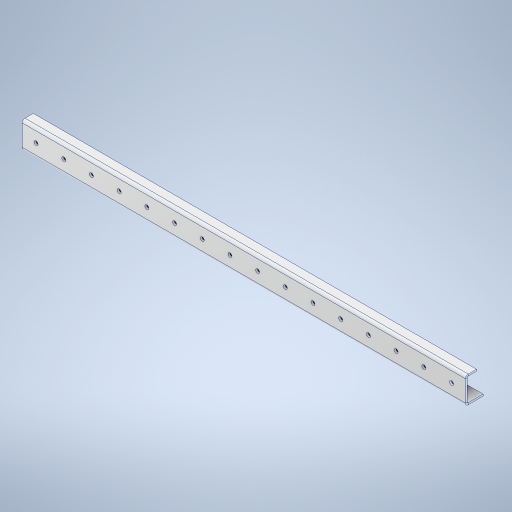
# Autodesk Inventor part: Gantry Stiffener
Saved by Autodesk Inventor 2024 (Build 280153000, 153)
## iProperties
Created: 2023-06-16
Part Number: Gantry Stiffener
Material: Aluminum 6061
Document SubType Name: Sheet Metal
Designer: Ishaan
Density: 2.7 g/cm^3
Appearance: Aluminum - Flat
Sheet Metal Rule: SendCutSend_Alu_1-16
Author: Ishaan
Autodesk Inventor part; units mm, degrees
ref_plane "YZ Plane" through (0, 0, 0) normal (1, 0, 0) x (0, 1, 0)
ref_plane "XZ Plane" through (0, 0, 0) normal (0, 1, 0) x (-1, 0, 0)
ref_plane "XY Plane" through (0, 0, 0) normal (0, 0, 1) x (1, 0, 0)
sketch "Sketch1" plane through (0, 0, 0) normal (0, 0, 1) x (1, 0, 0)
  line L0 (200, -12) -> (-200, -12)
  line L1 (-200, -12) -> (-200, 12)
  line L2 (-200, 12) -> (200, 12)
  line L3 (200, 12) -> (200, -12)
  line L4 (200, -12) -> (-200, 12) construction
  line L5 (-200, -12) -> (200, 12) construction
  point P0 (0, 0)
  dimension "d69" = 400
  dimension "d70" = 24
  constraints: 12 end point, 2 midpoint, 2 parallel, 1 horizontal, 1 perpendicular
  measures "d69" distance of L1.end L2.end
  measures "d70" distance of L0.end L1.end
extrude "Plate4" add sketch "Sketch1" along normal blind 1.6002
sketch "Sketch6" plane through (200, 10.3998, 1.6002) normal (0, 1, 0) x (-1, 0, 0)
  line L0 (400, 0) -> (0, 0)
  line L1 (0, 0) -> (0, -10)
  line L2 (0, -10) -> (400, -10)
  line L3 (400, -10) -> (400, 0)
  constraints: 6 end point, 1 horizontal, 1 perpendicular, 1 vertical
edge flange "Flange3" height 10 angle 90 thickness 1.6002 bend radius 0.889 thickness toward (0, 1, 0) relief tear relief width 1.6002 relief depth 0.8001 edges at (0, 12, 0) wall of the first edge with corners at (-200, 10.3998, 1.6002) (200, 10.3998, 1.6002) (200, 10.3998, -8.3998) (-200, 10.3998, -8.3998)
bend "Bend3"
corner "Corner3"
sketch "Sketch7" plane through (-200, -10.3998, 1.6002) normal (0, -1, 0) x (1, 0, 0)
  line L0 (400, 0) -> (0, 0)
  line L1 (0, 0) -> (0, -16)
  line L2 (0, -16) -> (400, -16)
  line L3 (400, -16) -> (400, 0)
  constraints: 6 end point, 1 horizontal, 1 perpendicular, 1 vertical
edge flange "Flange4" height 16 angle 90 thickness 1.6002 bend radius 0.889 thickness toward (0, -1, 0) relief tear relief width 1.6002 relief depth 0.8001 edges at (0, -12, 0) wall of the first edge with corners at (200, -10.3998, 1.6002) (-200, -10.3998, 1.6002) (-200, -10.3998, -14.3998) (200, -10.3998, -14.3998)
bend "Bend4"
corner "Corner4"
sketch "Sketch8" plane through (0, 0, 1.6002) normal (0, 0, 1) x (1, 0, 0)
  line L0 (-280, 0) -> (280, 0) construction
  line L1 (-187.5, 0) -> (187.5, 0) construction
  point P0 (0, 0)
  point P1 (-162.5, 0)
  point P2 (-137.5, 0)
  point P3 (-112.5, 0)
  point P4 (-87.5, 0)
  point P5 (-62.5, 0)
  point P6 (-37.5, 0)
  point P7 (-12.5, 0)
  point P8 (12.5, 0)
  point P9 (37.5, 0)
  point P10 (62.5, 0)
  point P11 (87.5, 0)
  point P12 (112.5, 0)
  point P13 (137.5, 0)
  point P14 (162.5, 0)
  dimension "d94" = 25
  constraints: 2 end point, 2 horizontal, 1 midpoint, 15 other
  measures "d94" distance of L1.start point (-162.5, 0)
hole "Hole3" at (-187.5, 0, 1.6002) at (-162.5, 0, 1.6002) at (-137.5, 0, 1.6002) at (-112.5, 0, 1.6002) at (-87.5, 0, 1.6002) at (-62.5, 0, 1.6002) at (-37.5, 0, 1.6002) at (-12.5, 0, 1.6002) at (12.5, 0, 1.6002) at (37.5, 0, 1.6002) at (62.5, 0, 1.6002) at (87.5, 0, 1.6002) at (112.5, 0, 1.6002) at (137.5, 0, 1.6002) at (162.5, 0, 1.6002) at (187.5, 0, 1.6002) direction (0, 0, -1) diameter 3.5 end through all
sketch "Sketch9" plane through (-200, -12, -14.3998) normal (0, -1, 0) x (1, 0, 0)
  line L0 (110, -6) -> (90, -6)
  line L1 (90, -6) -> (90, 13.5)
  line L2 (90, 13.5) -> (110, 13.5)
  line L3 (110, 13.5) -> (110, -6)
  line L4 (110, -6) -> (90, 13.5) construction
  line L5 (90, -6) -> (110, 13.5) construction
  line L6 (100, -4.3329) -> (93, -0.2915)
  line L7 (93, -0.2915) -> (93, 7.7915)
  line L8 (93, 7.7915) -> (100, 11.8329)
  line L9 (100, 11.8329) -> (107, 7.7915)
  line L10 (107, 7.7915) -> (107, -0.2915)
  line L11 (107, -0.2915) -> (100, -4.3329)
  line L12 (93, 7.7915) -> (100, 3.75)
  line L13 (100, 3.75) -> (107, 7.7915)
  line L14 (93, 2.4028) -> (100, -1.6386)
  line L15 (100, -1.6386) -> (107, 2.4028)
  line L16 (107, 3.75) -> (100, -0.2915)
  line L17 (100, -0.2915) -> (93, 3.75)
  line L18 (93, 6.4443) -> (100, 2.4028)
  line L19 (100, 2.4028) -> (107, 6.4443)
  line L20 (0, 16) -> (400, 16) projected
  line L21 (400, 13.5108) -> (0, 13.5108) projected
  line L22 (400, 0) -> (0, 0) projected
  line L23 (90, -6) -> (86.5359, 0)
  line L24 (400, 0) -> (0, 0) projected
  line L25 (110, -6) -> (113.4641, 0)
  line L26 (93, 3.75) -> (95.3333, 5.0972)
  line L27 (107, 3.75) -> (104.6667, 5.0972)
  line L28 (107, -0.2915) -> (104.6667, 1.0557)
  line L29 (93, -0.2915) -> (95.3333, 1.0557)
  point P0 (200, 14.3998)
  point P1 (200, 13.5108)
  point P2 (113.4641, 0)
  point P3 (100.5048, 0)
  point P4 (99.4952, 0)
  point P5 (107, 0)
  point P6 (102.8381, 0)
  point P7 (97.1619, 0)
  point P8 (93, 0)
  point P9 (93.5048, 0)
  point P10 (106.4952, 0)
  dimension "d106" = 20
  dimension "d107" = 19.5
  dimension "d110" = 2.3333
  dimension "d111" = 2.3333
  dimension "d112" = 1.1667
  dimension "d113" = 1.1667
  dimension "d114" = 14
  dimension "d115" = 22
  dimension "d116" = 100
  dimension "d117" = 120
  dimension "d118" = 120
  constraints: 52 end point, 12 parallel, 10 point on line, 5 midpoint, 4 vertical alignment, 1 coincident, 1 horizontal, 1 perpendicular, 1 vertical, 13 other
  measures "d106" distance of L1.end L2.end
  measures "d107" distance of L0.end L1.end
  measures "d110" distance between parallel lines of L17 L18
  measures "d111" distance between parallel lines of L6 L14
  measures "d112" distance between parallel lines of L14 L17
  measures "d113" distance between parallel lines of L12 L18
  measures "d114" distance between parallel lines of L10 L7
  measures "d115" distance between parallel lines of L0 L20
  measures "d116" horizontal distance of point (200, 13.511) L12.end
  measures "d117" angle of L0 L23
  measures "d118" angle of L0 L25
extrude "Extrusion5" add sketch "Sketch9" against normal up to surface (1.6002 mm away) contours L0 L1 L22 L7 L6 L11 L10 L3 | L3 L22 L25 | L23 L22 L1 | L10 L28 L22 | L22 L29 L7 | L11 L6 L29 L22 L14 L15 L28 | L15 L14 L22 L17 L16 | L16 L17 L22
extrude "Extrusion6" cut sketch "Sketch9" against normal up to surface (1.6002 mm away) contours L11 L6 L29 L22 L14 L15 L28 | L22 L15 L28 | L29 L14 L22 | L16 L22 L17 L26 L18 L19 L27 | L16 L17 L22 | L13 L12 L8 L9
fillet "Fillet4" radius 2 4 edges at (-86.5359, -11.1999, -14.3998) (-90, -11.1999, -20.3998) (-113.4641, -11.1999, -14.3998) (-110, -11.1999, -20.3998)
fillet "Fillet6" radius 0.6 6 edges at (-100, -11.1999, -10.6498) (-100, -11.1999, -2.5669) (-100, -11.1999, -14.6913) (-100, -11.1999, -16.0384) (-100, -11.1999, -11.997) (-100, -11.1999, -18.7327)
fillet "Fillet5" radius 0.3 10 edges at (-93, -11.1999, -10.6498) (-107, -11.1999, -10.6498) (-93, -11.1999, -14.6913) (-107, -11.1999, -14.6913) (-93, -11.1999, -6.6083) (-107, -11.1999, -6.6083) (-104.6667, -11.1999, -9.3026) (-104.6667, -11.1999, -13.3441) (-95.3333, -11.1999, -9.3026) (-95.3333, -11.1999, -13.3441)
equation "\"d104\" = Thickness"
equation "\"d111\" = d110"
equation "\"d112\" = 0.5 * d111"
equation "\"d113\" = 0.5 * d110"
equation "\"d118\" = d117"
equation "\"d71\" = Thickness"
equation "\"d72\" = BendReliefWidth"
equation "\"d73\" = BendReliefDepth"
equation "\"d74\" = MinimumRemnant"
equation "\"d75\" = TransitionRadius"
equation "\"d78\" = BendRadius"
equation "\"d79\" = CornerReliefSize"
equation "\"d80\" = GapSize"
equation "\"d81\" = JacobiRadiusSize"
equation "\"d82\" = BendReliefWidth"
equation "\"d83\" = BendReliefDepth"
equation "\"d84\" = MinimumRemnant"
equation "\"d85\" = TransitionRadius"
equation "\"d88\" = BendRadius"
equation "\"d89\" = CornerReliefSize"
equation "\"d90\" = GapSize"
equation "\"d91\" = JacobiRadiusSize"
equation "\"BendReliefWidth\" = Thickness"
equation "\"BendReliefDepth\" = 0.5 * Thickness"
equation "\"CornerReliefSize\" = 4 * Thickness"
equation "\"MinimumRemnant\" = 2 * Thickness"
equation "\"TransitionRadius\" = BendRadius"
equation "\"JacobiRadiusSize\" = BendRadius"
equation "\"GapSize\" = Thickness"
equation "\"Thickness\" = 1.6002"
equation "\"BendRadius\" = 0.889"
body "Solid2"
